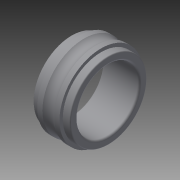
# Autodesk Inventor part: RF-2210X2HH_ir
Saved by Autodesk Inventor 2014 SP2 (Build 180246200, 246)
## iProperties
Created: 2019-07-25
Part Number: RF-2210X2HH_ir
Material: Generic
Catalog Web Link: www.cadenas.de
Description: Radial Flanged Ball Bearings (RF-Series/LF series) Metric ST ir-Radial Flanged Ball Bearings (RF-Series/LF series) Metric Shielded Type
Vendor: NMB
Document SubType Name: Modeling
Designer: psadmin
Manufacturer: NMB
Mass: 0.312147 g
Surface Area: 5.51818 cm^2
Volume: 0.312147 cm^3
Density: 1 g/cm^3
Appearance: PSOLRGB-192-192-192
Category: PARTsolutions
Company: NMB
Title: RF-2210X2HH_ir
Author: Cadenas PARTsolutions
Comments: Radial Flanged Ball Bearings (RF-Series/LF series) Metric Shielded Type
PSOL_IDENT_0: {$CADENAS_DATA\23d-libs\nmb\pbbp\radial_flanged_ball_bearings\rfbb_rflfs_m\rflf_shielded_ir.prj},227
PSOL_IDENT_1: {VTYP=3D},{NB=RF-2210X2HH_ir},{LINA=RF-2210X2HH_ir},{NN=Radial Flanged Ball Bearings (RF-Series/LF
PSOL_IDENT_2: series) Metric ST ir},{DATE=11.11.2013 05:13:45},{GEOMDATE=24.10.2013 10:33:00},{VERSION=},{LINEID=1
PSOL_IDENT_3: 560},{WBVAR=},{WBNUMERIC=}  {NB=RF-2210X2HH_ir},{LINA=RF-2210X2HH_ir},{KT=DUMMY},{IDNR=},{PN=RF-2210
PSOL_IDENT_4: X2HH},{SHLD=shielded},{FLANG=flanged},{SD=10.000},{D=22.000},{B=6.000},{SR=0.30},{BCZ=9},{DW=3.1750}
PSOL_IDENT_5: ,{LI=12.40},{LO=19.08},{D1=25.000},{C1=1.50},{D2=0.0},{C2=0.00},{COR=1273},{CR=1065},{PCD=16.000},{U=
PSOL_IDENT_6: 19.175},{W=12.825},{Y=1.588},{Z=1.588},{AA=18.858},{AC=1.20},{AD=0.000},{AF=0.00},{AQ=0.20},{AH=19.2
PSOL_IDENT_7: 8},{AI=12.60},{AJ=0.40}
NN: Radial Flanged Ball Bearings (RF-Series/LF series) Metric ST ir
NT: Radial Flanged Ball Bearings (RF-Series/LF series) Metric Shielded Type
NB: RF-2210X2HH_ir
NBSYN: $PN._ir
LINA: RF-2210X2HH_ir
PN: RF-2210X2HH
SHLD: shielded
FLANG: flanged
SD: 10
D: 22
B: 6
SR: 0.3
BCZ: 9
DW: 3.175
LI: 12.4
LO: 19.08
D1: 25
C1: 1.5
D2: 0
C2: 0
COR: 1273
CR: 1065
PCD: 16
U: 19.175
W: 12.825
Y: 1.588
Z: 1.588
AA: 18.858
AC: 1.2
AD: 0
AF: 0
AQ: 0.2
AH: 19.28
AI: 12.6
AJ: 0.4
SUPPLIER: NMB
ARTICLENO: RF-2210X2HH_ir
BOMINFO: RF-2210X2HH_ir
CREATOR: CADENAS GmbH
Autodesk Inventor part; units mm, degrees
ref_plane "YZ Plane" through (0, 0, 0) normal (1, 0, 0) x (0, 1, 0)
ref_plane "XZ Plane" through (0, 0, 0) normal (0, 1, 0) x (-1, 0, 0)
ref_plane "XY Plane" through (0, 0, 0) normal (0, 0, 1) x (1, 0, 0)
sketch "Sketch_6" plane through (0, 0, 0) normal (0, 0, 1) x (1, 0, 0)
  line L0 (6, 0) -> (0, 0)
  line L1 (0, 6.05) -> (0, 5.3)
  arc A0 (0, 5.3) -> (0.3, 5) centre (0.3, 5.3) ccw
  line L2 (0.3, 5) -> (5.7, 5)
  arc A1 (5.7, 5) -> (6, 5.3) centre (5.7, 5.3) ccw
  line L3 (6, 5.3) -> (6, 6.05)
  arc A2 (6, 6.05) -> (5.85, 6.2) centre (5.85, 6.05) ccw
  line L4 (5.85, 6.2) -> (4.8, 6.2)
  line L5 (4.8, 6.2) -> (4.8, 6.73)
  line L6 (4.8, 6.73) -> (3.9525, 6.73)
  arc A3 (2.0475, 6.73) -> (3.9525, 6.73) centre (3, 8) ccw
  line L7 (2.0475, 6.73) -> (1.2, 6.73)
  line L8 (1.2, 6.73) -> (1.2, 6.2)
  line L9 (1.2, 6.2) -> (0.15, 6.2)
  arc A4 (0.15, 6.2) -> (0, 6.05) centre (0.15, 6.05) ccw
  constraints: 20 end point, 10 point on circle, 5 centre point
revolve "Revolution1" add sketch "Sketch_6" angle 360 about axis through (6, 0, 0) along (1, 0, 0)
ref_plane "1_XY" through (3, 0, 0) normal (1, 0, 0) x (0, 0, -1)
ref_plane "1_YZ" through (3, 0, 0) normal (0, 0, -1) x (0, 1, 0)
ref_plane "1_ZX" through (3, 0, 0) normal (0, 1, 0) x (1, 0, 0)
ref_plane "Dummy_XY" through (0, 0, 0) normal (1, 0, 0) x (0, 0, -1)
ref_plane "Dummy_YZ" through (0, 0, 0) normal (0, 0, -1) x (0, 1, 0)
ref_plane "Dummy_ZX" through (0, 0, 0) normal (0, 1, 0) x (1, 0, 0)
ref_plane "shield1_XY" through (0.4, 0, 0) normal (1, 0, 0) x (0, 0, -1)
ref_plane "shield1_YZ" through (0.4, 0, 0) normal (0, 0, -1) x (0, 1, 0)
ref_plane "shield1_ZX" through (0.4, 0, 0) normal (0, 1, 0) x (1, 0, 0)
ref_plane "shield2_XY" through (5.6, 0, 0) normal (-1, 0, 0) x (0, 0, -1)
ref_plane "shield2_YZ" through (5.6, 0, 0) normal (0, 0, -1) x (0, -1, 0)
ref_plane "shield2_ZX" through (5.6, 0, 0) normal (0, -1, 0) x (-1, 0, 0)
body "Solid1"
